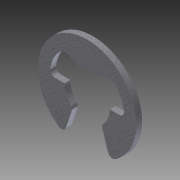
# Autodesk Inventor part: e clip .375in x ,039
Saved by Autodesk Inventor 2012 (Build 160160000, 160)
## iProperties
Created: 2011-12-24
Part Number: e clip .375in x ,039
Material: Default
Document SubType Name: Modeling
Designer: Bruce
Density: 1 g/cm^3
Author: Bruce
Autodesk Inventor part; units mm, degrees
ref_plane "YZ Plane" through (0, 0, 0) normal (1, 0, 0) x (0, 1, 0)
ref_plane "XZ Plane" through (0, 0, 0) normal (0, 1, 0) x (-1, 0, 0)
ref_plane "XY Plane" through (0, 0, 0) normal (0, 0, 1) x (1, 0, 0)
sketch "Sketch1" plane through (0, 0, 0) normal (0, 0, 1) x (1, 0, 0)
  arc A0 (2.4541, -2.964) -> (-1.2271, 3.6472) centre (0, 0) ccw
  arc A1 (3.9291, -7.4041) -> (8.3378, -0.86) centre (0, 0) ccw
  arc A2 (-3.9827, 4.9457) -> (-6.35, 0) centre (0, 0) ccw
  line L0 (1.2271, 3.6472) -> (3.9827, 4.9457)
  line L1 (-1.2271, 3.6472) -> (-3.9827, 4.9457)
  line L2 (3.8481, 0) -> (6.35, 0)
  line L3 (-3.8481, 0) -> (-6.35, 0)
  line L4 (2.4541, -2.964) -> (3.2154, -5.4758)
  line L5 (-2.4541, -2.964) -> (-3.2731, -5.4414)
  arc A3 (3.9827, 4.9457) -> (0.615, 6.3202) centre (0, 0) ccw
  arc A4 (0.615, 6.3202) -> (-0.3654, 6.3395) centre (0, 0) ccw
  arc A5 (6.35, 0) -> (6.3495, 0.0769) centre (0, 0) ccw
  line L6 (3.2154, -5.4758) -> (3.9291, -7.4041)
  arc A6 (-3.9291, -7.4041) -> (3.9291, -7.4041) centre (0, 0) ccw
  arc A7 (8.3378, -0.86) -> (-3.9291, -7.4041) centre (0, 0) ccw
  arc A8 (-2.4541, -2.964) -> (2.4541, -2.964) centre (0, 0) ccw
  arc A9 (-6.35, 0) -> (6.35, 0) centre (0, 0) ccw
  arc A10 (-3.8481, 0) -> (-2.4541, -2.964) centre (0, 0) ccw
  arc A11 (-1.2271, 3.6472) -> (-3.8481, 0) centre (0, 0) ccw
  arc A12 (-0.3654, 6.3395) -> (-3.9827, 4.9457) centre (0, 0) ccw
  arc A13 (6.3495, 0.0769) -> (3.9827, 4.9457) centre (0, 0) ccw
  line L7 (-3.2731, -5.4414) -> (-3.9291, -7.4041)
  dimension "d0" = 16.764
  dimension "d1" = 7.6962
  dimension "d2" = 12.7
  constraints: 39 point on circle, 16 end point, 14 centre point, 4 point on line, 3 coincident, 1 collinear, 1 horizontal
  measures "d0" diameter of A1
  measures "d1" diameter of A0
  measures "d2" diameter of A2
extrude "Extrusion1" add sketch "Sketch1" along normal blind 0.9906 contours A0 L2 A9 L4 | A9 A5 A13 A3 A4 A12 A2 L7 A7 A1 L6 | L5 A9 L3 A10 | A0 L1 A12 A4 A3 L0
fillet "Fillet1" radius 1.5875 2 edges at (-3.9827, 4.9457, 0.4953) (3.9827, 4.9457, 0.4953)
fillet "Fillet2" radius 0.7937 6 edges at (-6.35, 0, 0.4953) (6.35, 0, 0.4953) (-2.4541, -2.964, 0.4953) (2.4541, -2.964, 0.4953) (3.9291, -7.4041, 0.4953) (-3.9291, -7.4041, 0.4953)
body "Solid1"
